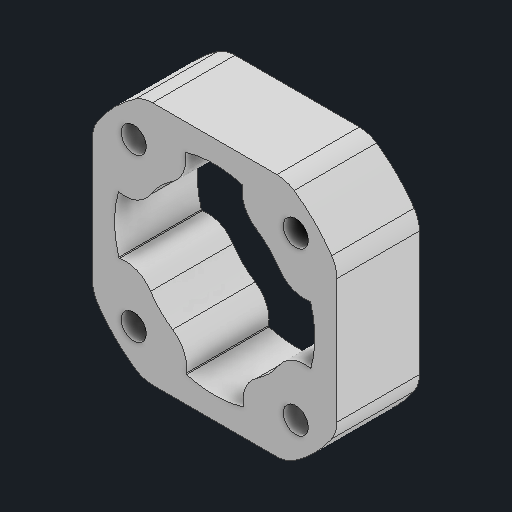
# Autodesk Inventor part: Test_block
Saved by Autodesk Inventor 2025.1 (Build 291241020, 241B)
## iProperties
Created: 2025-07-24
Part Number: Test_block
Material: 일반
Document SubType Name: Modeling
Designer: acalo
Density: 1 g/cm^3
Appearance: 기본값
Author: acalo
Autodesk Inventor part; units mm, degrees
ref_plane "YZ Plane" through (0, 0, 0) normal (1, 0, 0) x (0, 1, 0)
ref_plane "XZ Plane" through (0, 0, 0) normal (0, 1, 0) x (-1, 0, 0)
ref_plane "XY Plane" through (0, 0, 0) normal (0, 0, 1) x (1, 0, 0)
sketch "스케치1" plane through (0, 0, 0) normal (0, 0, 1) x (1, 0, 0)
  arc A0 (-1.531846, 18.436471) -> (1.531846, 18.436471) centre (0, 0) ccw
  circle A1 centre (10.606602, -10.606602) radius 1.65
  circle A2 centre (-10.606602, 10.606602) radius 1.65
  arc A3 (-12.136972, 5.585151) -> (-14.408043, 4.172324) centre (-12.486971, 3.616014) ccw
  arc A4 (-12.136972, 5.585151) -> (-10.10312, 6.475104) centre (-11.786973, 7.554288) ccw
  arc A5 (-6.573074, 10.039656) -> (-10.10312, 6.475104) centre (0, 0) ccw
  arc A6 (-6.573074, 10.039656) -> (-5.702947, 12.082069) centre (-7.668586, 11.712933) ccw
  arc A7 (-4.312278, 14.366776) -> (-5.702947, 12.082069) centre (-3.737307, 12.451206) ccw
  arc A8 (4.172324, 14.408043) -> (-4.312278, 14.366776) centre (0, 0) ccw
  arc A9 (5.585151, 12.136972) -> (4.172324, 14.408043) centre (3.616014, 12.486971) ccw
  arc A10 (5.585151, 12.136972) -> (6.475104, 10.10312) centre (7.554288, 11.786973) ccw
  arc A11 (10.039656, 6.573074) -> (6.475104, 10.10312) centre (0, 0) ccw
  arc A12 (10.039656, 6.573074) -> (12.082069, 5.702947) centre (11.712933, 7.668586) ccw
  arc A13 (14.366776, 4.312278) -> (12.082069, 5.702947) centre (12.451206, 3.737307) ccw
  arc A14 (14.408043, -4.172324) -> (14.366776, 4.312278) centre (0, 0) ccw
  arc A15 (12.136972, -5.585151) -> (14.408043, -4.172324) centre (12.486971, -3.616014) ccw
  arc A16 (12.136972, -5.585151) -> (10.10312, -6.475104) centre (11.786973, -7.554288) ccw
  arc A17 (6.573074, -10.039656) -> (10.10312, -6.475104) centre (0, 0) ccw
  arc A18 (6.573074, -10.039656) -> (5.702947, -12.082069) centre (7.668586, -11.712933) ccw
  arc A19 (4.312278, -14.366776) -> (5.702947, -12.082069) centre (3.737307, -12.451206) ccw
  arc A20 (-4.172324, -14.408043) -> (4.312278, -14.366776) centre (0, 0) ccw
  arc A21 (-5.585151, -12.136972) -> (-4.172324, -14.408043) centre (-3.616014, -12.486971) ccw
  arc A22 (-5.585151, -12.136972) -> (-6.475104, -10.10312) centre (-7.554288, -11.786973) ccw
  arc A23 (-10.039656, -6.573074) -> (-6.475104, -10.10312) centre (0, 0) ccw
  arc A24 (-10.039656, -6.573074) -> (-12.082069, -5.702947) centre (-11.712933, -7.668586) ccw
  arc A25 (-14.366776, -4.312278) -> (-12.082069, -5.702947) centre (-12.451206, -3.737307) ccw
  arc A26 (-14.408043, 4.172324) -> (-14.366776, -4.312278) centre (0, 0) ccw
  circle A27 centre (-10.606602, -10.606602) radius 1.65
  circle A28 centre (10.606602, 10.606602) radius 1.65
  circle A29 centre (0, 0) radius 18.5
  point P0 (0, 0)
  point P1 (0, 0)
  point P2 (1.531846, 18.436471)
  point P3 (-1.531846, 18.436471)
  constraints: 50 point on circle, 30 centre point, 1 coincident
extrude "돌출1" add sketch "스케치1" along normal blind 10.8
sketch "스케치2" plane through (0, 0, 0) normal (0, 0, -1) x (-1, 0, 0)
  circle A0 centre (0, 0) radius 10
  circle A1 centre (0, 0) radius 18.5
  circle A2 centre (-10.606602, 10.606602) radius 1.65
  circle A3 centre (10.606602, -10.606602) radius 1.65
  arc A4 (5.801316, 12.081591) -> (6.573074, 10.039656) centre (7.754884, 11.653138) ccw
  arc A5 (10.10312, 6.475104) -> (6.573074, 10.039656) centre (0, 0) ccw
  arc A6 (10.10312, 6.475104) -> (12.136972, 5.585151) centre (11.786973, 7.554288) ccw
  arc A7 (14.561385, 3.90838) -> (12.136972, 5.585151) centre (12.558013, 3.602834) ccw
  arc A8 (14.428046, -4.274984) -> (14.561385, 3.90838) centre (0.009899, 0.052713) ccw
  arc A9 (12.082069, -5.702947) -> (14.428046, -4.274984) centre (12.461105, -3.684594) ccw
  arc A10 (12.082069, -5.702947) -> (10.039656, -6.573074) centre (11.712933, -7.668586) ccw
  arc A11 (6.475104, -10.10312) -> (10.039656, -6.573074) centre (0, 0) ccw
  arc A12 (6.475104, -10.10312) -> (5.686974, -12.137467) centre (7.644162, -11.725865) ccw
  arc A13 (4.237586, -14.467309) -> (5.686974, -12.137467) centre (3.66688, -12.496523) ccw
  arc A14 (-4.27629, -14.425899) -> (4.237586, -14.467309) centre (0.050866, -0.009552) ccw
  arc A15 (-5.702947, -12.082069) -> (-4.27629, -14.425899) centre (-3.686441, -12.460759) ccw
  arc A16 (-5.702947, -12.082069) -> (-6.573074, -10.039656) centre (-7.668586, -11.712933) ccw
  arc A17 (-10.10312, -6.475104) -> (-6.573074, -10.039656) centre (0, 0) ccw
  arc A18 (-10.10312, -6.475104) -> (-12.13745, -5.683521) centre (-11.728021, -7.641164) ccw
  arc A19 (-14.465299, -4.235373) -> (-12.13745, -5.683521) centre (-12.496199, -3.665155) ccw
  arc A20 (-14.423894, 4.277511) -> (-14.465299, -4.235373) centre (-0.009228, -0.049141) ccw
  arc A21 (-12.082069, 5.702947) -> (-14.423894, 4.277511) centre (-12.460435, 3.688166) ccw
  arc A22 (-12.082069, 5.702947) -> (-10.039656, 6.573074) centre (-11.712933, 7.668586) ccw
  arc A23 (-6.475104, 10.10312) -> (-10.039656, 6.573074) centre (0, 0) ccw
  arc A24 (-6.475104, 10.10312) -> (-5.585151, 12.136972) centre (-7.554288, 11.786973) ccw
  arc A25 (-4.137004, 14.46482) -> (-5.585151, 12.136972) centre (-3.566786, 12.495721) ccw
  arc A26 (4.37588, 14.423416) -> (-4.137004, 14.46482) centre (0.049228, 0.00875) ccw
  arc A27 (5.801316, 12.081591) -> (4.37588, 14.423416) centre (3.786536, 12.459956) ccw
  circle A28 centre (10.606602, 10.606602) radius 1.65
  circle A29 centre (-10.606602, -10.606602) radius 1.65
  arc A30 (-12.441978, 3.786448) -> (-8.408212, 5.504949) centre (-11.712933, 7.668586) ccw
  arc A31 (-12.441978, 3.786448) -> (-12.556213, 3.716915) centre (-12.460435, 3.688166) ccw
  arc A32 (-12.556213, 3.716915) -> (-12.592253, -3.692971) centre (-0.009228, -0.049141) ccw
  arc A33 (-12.592253, -3.692971) -> (-12.478699, -3.763612) centre (-12.496199, -3.665155) ccw
  arc A34 (-8.402791, -5.51002) -> (-12.478699, -3.763612) centre (-11.728021, -7.641164) ccw
  arc A35 (-8.402791, -5.51002) -> (-5.503988, -8.406744) centre (0, 0) ccw
  arc A36 (-3.784723, -12.442302) -> (-5.503988, -8.406744) centre (-7.668586, -11.712933) ccw
  arc A37 (-3.784723, -12.442302) -> (-3.71519, -12.556537) centre (-3.686441, -12.460759) ccw
  arc A38 (-3.71519, -12.556537) -> (3.694696, -12.592577) centre (0.050866, -0.009552) ccw
  arc A39 (3.694696, -12.592577) -> (3.765337, -12.479023) centre (3.66688, -12.496523) ccw
  arc A40 (5.512089, -8.399187) -> (3.765337, -12.479023) centre (7.644162, -11.725865) ccw
  arc A41 (5.512089, -8.399187) -> (8.405172, -5.502958) centre (0, 0) ccw
  arc A42 (12.442649, -3.782876) -> (8.405172, -5.502958) centre (11.712933, -7.668586) ccw
  arc A43 (12.442649, -3.782876) -> (12.556884, -3.713343) centre (12.461105, -3.684594) ccw
  arc A44 (12.556884, -3.713343) -> (12.592924, 3.696543) centre (0.009899, 0.052713) ccw
  arc A45 (12.592924, 3.696543) -> (12.478528, 3.663514) centre (12.558013, 3.602834) ccw
  arc A46 (8.459885, 5.421953) -> (12.478528, 3.663514) centre (11.786973, 7.554288) ccw
  arc A47 (8.459885, 5.421953) -> (5.591495, 8.348797) centre (0, 0) ccw
  arc A48 (3.884818, 12.441499) -> (5.591495, 8.348797) centre (7.754884, 11.653138) ccw
  arc A49 (3.884818, 12.441499) -> (3.815284, 12.555735) centre (3.786536, 12.459956) ccw
  arc A50 (3.815284, 12.555735) -> (-3.594601, 12.591774) centre (0.049228, 0.00875) ccw
  arc A51 (-3.594601, 12.591774) -> (-3.665243, 12.478221) centre (-3.566786, 12.495721) ccw
  arc A52 (-5.4229, 8.461363) -> (-3.665243, 12.478221) centre (-7.554288, 11.786973) ccw
  arc A53 (-5.4229, 8.461363) -> (-8.408212, 5.504949) centre (0, 0) ccw
  point P0 (-8.450044, 5.532337)
  point P1 (-5.449879, 8.503459)
  point P2 (5.532337, 8.450044)
  point P3 (8.503459, 5.449879)
  point P4 (8.450044, -5.532337)
  point P5 (5.449879, -8.503459)
  point P6 (-5.532337, -8.450044)
  point P7 (-8.503459, -5.449879)
  dimension "d2" = 20
  dimension "d3" = 1.95
  constraints: 96 point on circle, 82 centre point, 1 coincident, 4 other
  measures "d2" diameter of A0
  measures "d3" radial gap between concentric circles of A23 A53
extrude "돌출2" add sketch "스케치2" against normal up to surface (10.8 mm away) contours A4 A5 A6 A7 A8 A9 A10 A11 A12 A13 A14 A15 A16 A17 A18 A19 A20 A21 A22 A23 A24 A25 A26 A27
sketch "스케치3" plane through (0, 0, 0) normal (0, 0, -1) x (-1, 0, 0)
  line L0 (-16, 16) -> (16, 16)
  line L1 (16, 16) -> (16, -16)
  line L2 (16, -16) -> (-16, -16)
  line L3 (-16, -16) -> (-16, 16)
  line L4 (-16, 16) -> (16, -16) construction
  line L5 (16, 16) -> (-16, -16) construction
  circle A0 centre (0, 0) radius 18.5
  circle A1 centre (-10.606602, 10.606602) radius 1.65
  circle A2 centre (10.606602, -10.606602) radius 1.65
  circle A3 centre (10.606602, 10.606602) radius 1.65
  circle A4 centre (-10.606602, -10.606602) radius 1.65
  point P0 (0, 0)
  point P1 (-9.287088, -16)
  point P2 (9.287088, -16)
  point P3 (16, 9.287088)
  point P4 (16, -9.287088)
  point P5 (9.287088, 16)
  point P6 (-9.287088, 16)
  point P7 (-16, 9.287088)
  point P8 (-16, -9.287088)
  dimension "d6" = 32
  dimension "d7" = 32
  constraints: 12 end point, 2 midpoint, 2 parallel, 1 horizontal, 1 perpendicular
  measures "d6" distance of L1.end L2.end
  measures "d7" distance of L0.end L1.end
extrude "돌출3" cut sketch "스케치3" against normal through all contours A0 L0 | L3 A0 | A0 L1 | L2 A0
fillet "모깎기1" radius 4 8 edges at (16, 9.2871, 5.4) (9.2871, 16, 5.4) (16, -9.2871, 5.4) (9.2871, -16, 5.4) (-9.2871, -16, 5.4) (-16, -9.2871, 5.4) (-16, 9.2871, 5.4) (-9.2871, 16, 5.4)
